Autodesk Fusion 360 part; units mm, degrees
(part 3 of 4)
  line L1469 (33.9941, -8.3096) -> (33.7624, -8.35)
  line L1470 (33.7624, -8.35) -> (33.6779, -8.255)
  line L1471 (33.6779, -8.255) -> (33.6779, -6.1823)
  line L1472 (5.5809, 13.4818) -> (5.5809, 13.4818)
  line L1473 (35.5029, -8.255) -> (35.5248, -6.0186)
  line L1474 (35.5248, -6.0186) -> (35.7566, -5.9782)
  line L1475 (35.7566, -5.9782) -> (35.8411, -6.0732)
  line L1476 (35.8411, -6.0732) -> (35.8411, -7.055)
  line L1477 (35.8411, -7.055) -> (36.8528, -7.055)
  line L1478 (36.8528, -7.055) -> (36.8747, -6.0186)
  line L1479 (36.8747, -6.0186) -> (37.1065, -5.9782)
  line L1480 (37.1065, -5.9782) -> (37.191, -6.0732)
  line L1481 (37.191, -6.0732) -> (37.1691, -8.3096)
  line L1482 (37.1691, -8.3096) -> (36.9374, -8.35)
  line L1483 (36.9374, -8.35) -> (36.8528, -8.255)
  line L1484 (36.8528, -8.255) -> (36.8528, -7.2732)
  line L1485 (36.8528, -7.2732) -> (35.8411, -7.2732)
  line L1486 (35.8411, -7.2732) -> (35.8192, -8.3096)
  line L1487 (35.8192, -8.3096) -> (35.5875, -8.35)
  line L1488 (35.5875, -8.35) -> (35.5029, -8.255)
  line L1489 (7.406, 11.4091) -> (7.406, 11.4091)
  line L1490 (38.9963, -7.375) -> (39.1977, -7.2732)
  line L1491 (39.1977, -7.2732) -> (39.2415, -7.1641)
  line L1492 (39.2415, -7.1641) -> (39.2304, -6.3429)
  line L1493 (39.2304, -6.3429) -> (39.1071, -6.2265)
  line L1494 (39.1071, -6.2265) -> (38.9033, -6.1823)
  line L1495 (38.9033, -6.1823) -> (38.3397, -6.1823)
  line L1496 (38.3397, -6.1823) -> (38.3178, -8.3096)
  line L1497 (38.3178, -8.3096) -> (38.0861, -8.35)
  line L1498 (38.0861, -8.35) -> (38.0015, -8.255)
  line L1499 (38.0015, -8.255) -> (38.0234, -6.0186)
  line L1500 (38.0234, -6.0186) -> (38.1706, -5.9641)
  line L1501 (38.1706, -5.9641) -> (39.0804, -5.9783)
  line L1502 (39.0804, -5.9783) -> (39.3126, -6.0531)
  line L1503 (39.3126, -6.0531) -> (39.4914, -6.1835)
  line L1504 (39.4914, -6.1835) -> (39.5576, -6.2862)
  line L1505 (39.5576, -6.2862) -> (39.5797, -6.4005)
  line L1506 (39.5797, -6.4005) -> (39.5742, -7.2226)
  line L1507 (39.5742, -7.2226) -> (39.5304, -7.3309)
  line L1508 (39.5304, -7.3309) -> (39.2528, -7.5386)
  line L1509 (39.2528, -7.5386) -> (39.684, -8.2877)
  line L1510 (39.684, -8.2877) -> (39.4726, -8.3605)
  line L1511 (39.4726, -8.3605) -> (39.3711, -8.3041)
  line L1512 (39.3711, -8.3041) -> (38.8709, -7.4657)
  line L1513 (38.8709, -7.4657) -> (38.9963, -7.375)
  line L1514 (10.8994, 12.2891) -> (10.8994, 12.2891)
  line L1515 (40.641, -8.255) -> (40.6629, -6.0186)
  line L1516 (40.6629, -6.0186) -> (40.8101, -5.9641)
  line L1517 (40.8101, -5.9641) -> (42.0036, -5.9959)
  line L1518 (42.0036, -5.9959) -> (42.0474, -6.1011)
  line L1519 (42.0474, -6.1011) -> (41.8838, -6.1823)
  line L1520 (41.8838, -6.1823) -> (40.9792, -6.1823)
  line L1521 (40.9792, -6.1823) -> (40.9792, -7.055)
  line L1522 (40.9792, -7.055) -> (41.8317, -7.0868)
  line L1523 (41.8317, -7.0868) -> (41.8755, -7.1929)
  line L1524 (41.8755, -7.1929) -> (41.7119, -7.2732)
  line L1525 (41.7119, -7.2732) -> (40.9792, -7.2732)
  line L1526 (40.9792, -7.2732) -> (40.9792, -8.1459)
  line L1527 (40.9792, -8.1459) -> (42.0036, -8.1777)
  line L1528 (42.0036, -8.1777) -> (42.0474, -8.2829)
  line L1529 (42.0474, -8.2829) -> (41.8838, -8.3641)
  line L1530 (41.8838, -8.3641) -> (40.6903, -8.3323)
  line L1531 (40.6903, -8.3323) -> (40.641, -8.255)
  line L1532 (12.544, 11.4091) -> (12.544, 11.4091)
  line L1533 (43.141, -8.255) -> (43.1629, -6.0186)
  line L1534 (43.1629, -6.0186) -> (43.3101, -5.9641)
  line L1535 (43.3101, -5.9641) -> (44.5036, -5.9959)
  line L1536 (44.5036, -5.9959) -> (44.5474, -6.1011)
  line L1537 (44.5474, -6.1011) -> (44.3838, -6.1823)
  line L1538 (44.3838, -6.1823) -> (43.4792, -6.1823)
  line L1539 (43.4792, -6.1823) -> (43.4792, -7.055)
  line L1540 (43.4792, -7.055) -> (44.3317, -7.0868)
  line L1541 (44.3317, -7.0868) -> (44.3755, -7.1929)
  line L1542 (44.3755, -7.1929) -> (44.2119, -7.2732)
  line L1543 (44.2119, -7.2732) -> (43.4792, -7.2732)
  line L1544 (43.4792, -7.2732) -> (43.4792, -8.1459)
  line L1545 (43.4792, -8.1459) -> (44.5036, -8.1777)
  line L1546 (44.5036, -8.1777) -> (44.5474, -8.2829)
  line L1547 (44.5474, -8.2829) -> (44.3838, -8.3641)
  line L1548 (44.3838, -8.3641) -> (43.1903, -8.3323)
  line L1549 (43.1903, -8.3323) -> (43.141, -8.255)
  line L1550 (15.044, 11.4091) -> (15.044, 11.4091)
  line L1551 (46.1751, -7.6132) -> (45.5068, -6.0444)
  line L1552 (45.5068, -6.0444) -> (45.6907, -5.965)
  line L1553 (45.6907, -5.965) -> (45.8284, -6.0368)
  line L1554 (45.8284, -6.0368) -> (46.347, -7.215)
  line L1555 (46.347, -7.215) -> (46.9106, -5.995)
  line L1556 (46.9106, -5.995) -> (47.1459, -5.9959)
  line L1557 (47.1459, -5.9959) -> (47.184, -6.1168)
  line L1558 (47.184, -6.1168) -> (46.5132, -7.615)
  line L1559 (46.5132, -7.615) -> (46.4913, -8.3096)
  line L1560 (46.4913, -8.3096) -> (46.2615, -8.35)
  line L1561 (46.2615, -8.35) -> (46.1751, -8.255)
  line L1562 (46.1751, -8.255) -> (46.1751, -7.6132)
  line L1563 (18.0781, 12.0509) -> (18.0781, 12.0509)
  line L1564 (48.4792, -7.055) -> (49.3317, -7.0868)
  line L1565 (49.3317, -7.0868) -> (49.3755, -7.1929)
  line L1566 (49.3755, -7.1929) -> (49.2119, -7.2732)
  line L1567 (49.2119, -7.2732) -> (48.4792, -7.2732)
  line L1568 (48.4792, -7.2732) -> (48.4573, -8.3096)
  line L1569 (48.4573, -8.3096) -> (48.2256, -8.35)
  line L1570 (48.2256, -8.35) -> (48.141, -8.255)
  line L1571 (48.141, -8.255) -> (48.1629, -6.0186)
  line L1572 (48.1629, -6.0186) -> (48.3101, -5.9641)
  line L1573 (48.3101, -5.9641) -> (49.5036, -5.9959)
  line L1574 (49.5036, -5.9959) -> (49.5474, -6.1011)
  line L1575 (49.5474, -6.1011) -> (49.3838, -6.1823)
  line L1576 (49.3838, -6.1823) -> (48.4792, -6.1823)
  line L1577 (48.4792, -6.1823) -> (48.4792, -7.055)
  line L1578 (20.3822, 12.6091) -> (20.3822, 12.6091)
  line L1579 (51.1779, -8.255) -> (51.1998, -6.0186)
  line L1580 (51.1998, -6.0186) -> (51.4315, -5.9782)
  line L1581 (51.4315, -5.9782) -> (51.5161, -6.0732)
  line L1582 (51.5161, -6.0732) -> (51.4941, -8.3096)
  line L1583 (51.4941, -8.3096) -> (51.2624, -8.35)
  line L1584 (51.2624, -8.35) -> (51.1779, -8.255)
  line L1585 (23.0809, 11.4091) -> (23.0809, 11.4091)
  line L1586 (53.4792, -7.055) -> (54.3317, -7.0868)
  line L1587 (54.3317, -7.0868) -> (54.3755, -7.1929)
  line L1588 (54.3755, -7.1929) -> (54.2119, -7.2732)
  line L1589 (54.2119, -7.2732) -> (53.4792, -7.2732)
  line L1590 (53.4792, -7.2732) -> (53.4573, -8.3096)
  line L1591 (53.4573, -8.3096) -> (53.2256, -8.35)
  line L1592 (53.2256, -8.35) -> (53.141, -8.255)
  line L1593 (53.141, -8.255) -> (53.1629, -6.0186)
  line L1594 (53.1629, -6.0186) -> (53.3101, -5.9641)
  line L1595 (53.3101, -5.9641) -> (54.5036, -5.9959)
  line L1596 (54.5036, -5.9959) -> (54.5474, -6.1011)
  line L1597 (54.5474, -6.1011) -> (54.3838, -6.1823)
  line L1598 (54.3838, -6.1823) -> (53.4792, -6.1823)
  line L1599 (53.4792, -6.1823) -> (53.4792, -7.055)
  line L1600 (25.3822, 12.6091) -> (25.3822, 12.6091)
  line L1601 (55.2789, -6.0968) -> (55.3424, -5.9862)
  line L1602 (55.3424, -5.9862) -> (55.6142, -6.055)
  line L1603 (55.6142, -6.055) -> (56.347, -7.8277)
  line L1604 (56.347, -7.8277) -> (57.1304, -5.995)
  line L1605 (57.1304, -5.995) -> (57.3686, -5.9959)
  line L1606 (57.3686, -5.9959) -> (57.4151, -6.0968)
  line L1607 (57.4151, -6.0968) -> (56.4681, -8.3314)
  line L1608 (56.4681, -8.3314) -> (56.1852, -8.2809)
  line L1609 (56.1852, -8.2809) -> (55.2789, -6.0968)
  line L1610 (27.1819, 13.5673) -> (27.1819, 13.5673)
  line L1611 (58.8892, -8.1459) -> (59.1257, -8.0853)
  line L1612 (59.1257, -8.0853) -> (59.2648, -7.9696)
  line L1613 (59.2648, -7.9696) -> (59.2979, -7.8586)
  line L1614 (59.2979, -7.8586) -> (59.2942, -6.4341)
  line L1615 (59.2942, -6.4341) -> (59.239, -6.3285)
  line L1616 (59.239, -6.3285) -> (59.0712, -6.2203)
  line L1617 (59.0712, -6.2203) -> (58.847, -6.1823)
  line L1618 (58.847, -6.1823) -> (58.3961, -6.1823)
  line L1619 (58.3961, -6.1823) -> (58.3741, -8.3096)
  line L1620 (58.3741, -8.3096) -> (58.1424, -8.35)
  line L1621 (58.1424, -8.35) -> (58.0579, -8.255)
  line L1622 (58.0579, -8.255) -> (58.0798, -6.0186)
  line L1623 (58.0798, -6.0186) -> (58.227, -5.9641)
  line L1624 (58.227, -5.9641) -> (58.9533, -5.9682)
  line L1625 (58.9533, -5.9682) -> (59.2403, -6.0304)
  line L1626 (59.2403, -6.0304) -> (59.4756, -6.1646)
  line L1627 (59.4756, -6.1646) -> (59.5783, -6.2777)
  line L1628 (59.5783, -6.2777) -> (59.6296, -6.4046)
  line L1629 (59.6296, -6.4046) -> (59.6296, -7.9272)
  line L1630 (59.6296, -7.9272) -> (59.5783, -8.0536)
  line L1631 (59.5783, -8.0536) -> (59.4756, -8.166)
  line L1632 (59.4756, -8.166) -> (59.259, -8.293)
  line L1633 (59.259, -8.293) -> (59.0073, -8.3565)
  line L1634 (59.0073, -8.3565) -> (58.7562, -8.3096)
  line L1635 (58.7562, -8.3096) -> (58.7568, -8.2009)
  line L1636 (58.7568, -8.2009) -> (58.8892, -8.1459)
  line L1637 (30.7923, 11.5182) -> (30.7923, 11.5182)
  line L1638 (30.641, -11.255) -> (30.6629, -9.0186)
  line L1639 (30.6629, -9.0186) -> (30.8101, -8.9641)
  line L1640 (30.8101, -8.9641) -> (32.0036, -8.9959)
  line L1641 (32.0036, -8.9959) -> (32.0474, -9.1011)
  line L1642 (32.0474, -9.1011) -> (31.8838, -9.1823)
  line L1643 (31.8838, -9.1823) -> (30.9792, -9.1823)
  line L1644 (30.9792, -9.1823) -> (30.9792, -10.055)
  line L1645 (30.9792, -10.055) -> (31.8317, -10.0868)
  line L1646 (31.8317, -10.0868) -> (31.8755, -10.1929)
  line L1647 (31.8755, -10.1929) -> (31.7119, -10.2732)
  line L1648 (31.7119, -10.2732) -> (30.9792, -10.2732)
  line L1649 (30.9792, -10.2732) -> (30.9792, -11.1459)
  line L1650 (30.9792, -11.1459) -> (32.0036, -11.1777)
  line L1651 (32.0036, -11.1777) -> (32.0474, -11.2829)
  line L1652 (32.0474, -11.2829) -> (31.8838, -11.3641)
  line L1653 (31.8838, -11.3641) -> (30.6903, -11.3323)
  line L1654 (30.6903, -11.3323) -> (30.641, -11.255)
  line L1655 (2.544, 8.4091) -> (2.544, 8.4091)
  line L1656 (33.6779, -11.255) -> (33.6998, -9.0186)
  line L1657 (33.6998, -9.0186) -> (33.9315, -8.9782)
  line L1658 (33.9315, -8.9782) -> (34.0161, -9.0732)
  line L1659 (34.0161, -9.0732) -> (33.9941, -11.3096)
  line L1660 (33.9941, -11.3096) -> (33.7624, -11.35)
  line L1661 (33.7624, -11.35) -> (33.6779, -11.255)
  line L1662 (5.5809, 8.4091) -> (5.5809, 8.4091)
  line L1663 (36.9045, -9.118) -> (36.9463, -9.2215)
  line L1664 (36.9463, -9.2215) -> (36.7415, -9.297)
  line L1665 (36.7415, -9.297) -> (36.4641, -9.1904)
  line L1666 (36.4641, -9.1904) -> (36.1753, -9.2017)
  line L1667 (36.1753, -9.2017) -> (35.9927, -9.2938)
  line L1668 (35.9927, -9.2938) -> (35.9175, -9.392)
  line L1669 (35.9175, -9.392) -> (35.9067, -10.9014)
  line L1670 (35.9067, -10.9014) -> (35.9604, -11.0054)
  line L1671 (35.9604, -11.0054) -> (36.1244, -11.1119)
  line L1672 (36.1244, -11.1119) -> (36.347, -11.1493)
  line L1673 (36.347, -11.1493) -> (36.7908, -11.1493)
  line L1674 (36.7908, -11.1493) -> (36.7908, -10.3261)
  line L1675 (36.7908, -10.3261) -> (36.4795, -10.2712)
  line L1676 (36.4795, -10.2712) -> (36.4795, -10.165)
  line L1677 (36.4795, -10.165) -> (36.6244, -10.1113)
  line L1678 (36.6244, -10.1113) -> (37.091, -10.1534)
  line L1679 (37.091, -10.1534) -> (37.1237, -10.2187)
  line L1680 (37.1237, -10.2187) -> (37.1021, -11.3092)
  line L1681 (37.1021, -11.3092) -> (36.9573, -11.3641)
  line L1682 (36.9573, -11.3641) -> (36.2423, -11.36)
  line L1683 (36.2423, -11.36) -> (35.9598, -11.2993)
  line L1684 (35.9598, -11.2993) -> (35.7282, -11.1679)
  line L1685 (35.7282, -11.1679) -> (35.6271, -11.0569)
  line L1686 (35.6271, -11.0569) -> (35.5766, -10.9323)
  line L1687 (35.5766, -10.9323) -> (35.5766, -9.3977)
  line L1688 (35.5766, -9.3977) -> (35.6271, -9.2728)
  line L1689 (35.6271, -9.2728) -> (35.7282, -9.1615)
  line L1690 (35.7282, -9.1615) -> (35.9598, -9.0293)
  line L1691 (35.9598, -9.0293) -> (36.2423, -8.9682)
  line L1692 (36.2423, -8.9682) -> (36.5519, -8.9812)
  line L1693 (36.5519, -8.9812) -> (36.9045, -9.118)
  line L1694 (8.8076, 10.5461) -> (8.8076, 10.5461)
  line L1695 (38.0029, -11.255) -> (38.0248, -9.0186)
  line L1696 (38.0248, -9.0186) -> (38.2566, -8.9782)
  line L1697 (38.2566, -8.9782) -> (38.3411, -9.0732)
  line L1698 (38.3411, -9.0732) -> (38.3411, -10.055)
  line L1699 (38.3411, -10.055) -> (39.3528, -10.055)
  line L1700 (39.3528, -10.055) -> (39.3747, -9.0186)
  line L1701 (39.3747, -9.0186) -> (39.6065, -8.9782)
  line L1702 (39.6065, -8.9782) -> (39.691, -9.0732)
  line L1703 (39.691, -9.0732) -> (39.6691, -11.3096)
  line L1704 (39.6691, -11.3096) -> (39.4374, -11.35)
  line L1705 (39.4374, -11.35) -> (39.3528, -11.255)
  line L1706 (39.3528, -11.255) -> (39.3528, -10.2732)
  line L1707 (39.3528, -10.2732) -> (38.3411, -10.2732)
  line L1708 (38.3411, -10.2732) -> (38.3192, -11.3096)
  line L1709 (38.3192, -11.3096) -> (38.0875, -11.35)
  line L1710 (38.0875, -11.35) -> (38.0029, -11.255)
  line L1711 (9.906, 8.4091) -> (9.906, 8.4091)
  line L1712 (41.1779, -9.1823) -> (40.5921, -9.1395)
  line L1713 (40.5921, -9.1395) -> (40.5702, -9.0311)
  line L1714 (40.5702, -9.0311) -> (40.727, -8.9641)
  line L1715 (40.727, -8.9641) -> (42.0867, -8.9959)
  line L1716 (42.0867, -8.9959) -> (42.1306, -9.102)
  line L1717 (42.1306, -9.102) -> (41.967, -9.1823)
  line L1718 (41.967, -9.1823) -> (41.5161, -9.1823)
  line L1719 (41.5161, -9.1823) -> (41.4941, -11.3096)
  line L1720 (41.4941, -11.3096) -> (41.2624, -11.35)
  line L1721 (41.2624, -11.35) -> (41.1779, -11.255)
  line L1722 (41.1779, -11.255) -> (41.1779, -9.1823)
  line L1723 (13.0809, 10.4818) -> (13.0809, 10.4818)
  line L1724 (45.3536, -9.0968) -> (44.5749, -11.3314)
  line L1725 (44.5749, -11.3314) -> (44.3768, -11.3414)
  line L1726 (44.3768, -11.3414) -> (44.3187, -11.2696)
  line L1727 (44.3187, -11.2696) -> (43.847, -9.895)
  line L1728 (43.847, -9.895) -> (43.3321, -11.3314)
  line L1729 (43.3321, -11.3314) -> (43.134, -11.3414)
  line L1730 (43.134, -11.3414) -> (43.0734, -11.2696)
  line L1731 (43.0734, -11.2696) -> (42.3489, -9.0311)
  line L1732 (42.3489, -9.0311) -> (42.549, -8.9718)
  line L1733 (42.549, -8.9718) -> (42.6422, -9.055)
  line L1734 (42.6422, -9.055) -> (43.2256, -10.7877)
  line L1735 (43.2256, -10.7877) -> (43.7442, -9.3568)
  line L1736 (43.7442, -9.3568) -> (43.9535, -9.3586)
  line L1737 (43.9535, -9.3586) -> (44.0093, -9.4368)
  line L1738 (44.0093, -9.4368) -> (44.4684, -10.7877)
  line L1739 (44.4684, -10.7877) -> (45.0974, -8.995)
  line L1740 (45.0974, -8.995) -> (45.3117, -8.9959)
  line L1741 (45.3117, -8.9959) -> (45.3536, -9.0968)
  line L1742 (17.2566, 10.5673) -> (17.2566, 10.5673)
  line L1743 (46.6117, -9.173) -> (46.5159, -9.0749)
  line L1744 (46.5159, -9.0749) -> (46.6403, -8.9694)
  line L1745 (46.6403, -8.9694) -> (46.9045, -9.0495)
  line L1746 (46.9045, -9.0495) -> (47.0328, -9.1557)
  line L1747 (47.0328, -9.1557) -> (47.1098, -9.2756)
  line L1748 (47.1098, -9.2756) -> (47.1355, -9.4092)
  line L1749 (47.1355, -9.4092) -> (47.129, -10.9875)
  line L1750 (47.129, -10.9875) -> (47.0777, -11.1143)
  line L1751 (47.0777, -11.1143) -> (46.9751, -11.2273)
  line L1752 (46.9751, -11.2273) -> (46.662, -11.3632)
  line L1753 (46.662, -11.3632) -> (46.5173, -11.2693)
  line L1754 (46.5173, -11.2693) -> (46.7644, -11.0303)
  line L1755 (46.7644, -11.0303) -> (46.7975, -10.919)
  line L1756 (46.7975, -10.919) -> (46.7939, -9.3702)
  line L1757 (46.7939, -9.3702) -> (46.7387, -9.2647)
  line L1758 (46.7387, -9.2647) -> (46.6117, -9.173)
  line L1759 (18.5147, 10.4911) -> (18.5147, 10.4911)
  line L1760 (45.9105, -8.9841) -> (46.1561, -9.0198)
  line L1761 (46.1561, -9.0198) -> (46.1567, -9.1272)
  line L1762 (46.1567, -9.1272) -> (45.9552, -9.2647)
  line L1763 (45.9552, -9.2647) -> (45.9001, -9.3702)
  line L1764 (45.9001, -9.3702) -> (45.9001, -10.958)
  line L1765 (45.9001, -10.958) -> (45.9552, -11.0635)
  line L1766 (45.9552, -11.0635) -> (46.1766, -11.2385)
  line L1767 (46.1766, -11.2385) -> (46.0916, -11.3482)
  line L1768 (46.0916, -11.3482) -> (45.7894, -11.2787)
  line L1769 (45.7894, -11.2787) -> (45.6611, -11.1725)
  line L1770 (45.6611, -11.1725) -> (45.5841, -11.0526)
  line L1771 (45.5841, -11.0526) -> (45.5585, -10.919)
  line L1772 (45.5585, -10.919) -> (45.5649, -9.3407)
  line L1773 (45.5649, -9.3407) -> (45.6162, -9.2139)
  line L1774 (45.6162, -9.2139) -> (45.7188, -9.1009)
  line L1775 (45.7188, -9.1009) -> (45.9105, -8.9841)
  line L1776 (17.8135, 10.68) -> (17.8135, 10.68)
  line L1777 (48.2238, -11.2001) -> (48.1749, -11.1029)
  line L1778 (48.1749, -11.1029) -> (48.344, -11.0167)
  line L1779 (48.344, -11.0167) -> (48.7119, -11.1462)
  line L1780 (48.7119, -11.1462) -> (48.9964, -11.1178)
  line L1781 (48.9964, -11.1178) -> (49.1604, -11.0206)
  line L1782 (49.1604, -11.0206) -> (49.2296, -10.8598)
  line L1783 (49.2296, -10.8598) -> (49.2144, -10.76)
  line L1784 (49.2144, -10.76) -> (49.0923, -10.5437)
  line L1785 (49.0923, -10.5437) -> (48.8481, -10.305)
  line L1786 (48.8481, -10.305) -> (48.5132, -10.0492)
  line L1787 (48.5132, -10.0492) -> (48.2702, -9.8035)
  line L1788 (48.2702, -9.8035) -> (48.1488, -9.5719)
  line L1789 (48.1488, -9.5719) -> (48.1336, -9.4332)
  line L1790 (48.1336, -9.4332) -> (48.1703, -9.3033)
  line L1791 (48.1703, -9.3033) -> (48.2551, -9.1886)
  line L1792 (48.2551, -9.1886) -> (48.4626, -9.051)
  line L1793 (48.4626, -9.051) -> (48.7097, -8.978)
  line L1794 (48.7097, -8.978) -> (49.0426, -8.9715)
  line L1795 (49.0426, -8.9715) -> (49.3153, -9.0409)
  line L1796 (49.3153, -9.0409) -> (49.5179, -9.1947)
  line L1797 (49.5179, -9.1947) -> (49.3954, -9.3066)
  line L1798 (49.3954, -9.3066) -> (49.035, -9.19)
  line L1799 (49.035, -9.19) -> (48.739, -9.1951)
  line L1800 (48.739, -9.1951) -> (48.5652, -9.2755)
  line L1801 (48.5652, -9.2755) -> (48.4825, -9.3703)
  line L1802 (48.4825, -9.3703) -> (48.4616, -9.4596)
  line L1803 (48.4616, -9.4596) -> (48.5232, -9.6395)
  line L1804 (48.5232, -9.6395) -> (48.7082, -9.8523)
  line L1805 (48.7082, -9.8523) -> (49.1826, -10.2267)
  line L1806 (49.1826, -10.2267) -> (49.4244, -10.4811)
  line L1807 (49.4244, -10.4811) -> (49.5452, -10.7311)
  line L1808 (49.5452, -10.7311) -> (49.5576, -10.8933)
  line L1809 (49.5576, -10.8933) -> (49.5209, -11.0232)
  line L1810 (49.5209, -11.0232) -> (49.4361, -11.1378)
  line L1811 (49.4361, -11.1378) -> (49.2286, -11.2759)
  line L1812 (49.2286, -11.2759) -> (48.9803, -11.35)
  line L1813 (48.9803, -11.35) -> (48.6486, -11.3561)
  line L1814 (48.6486, -11.3561) -> (48.3759, -11.2857)
  line L1815 (48.3759, -11.2857) -> (48.2238, -11.2001)
  line L1816 (20.1268, 8.464) -> (20.1268, 8.464)
  line L1817 (51.1779, -11.255) -> (51.1998, -9.0186)
  line L1818 (51.1998, -9.0186) -> (51.4315, -8.9782)
  line L1819 (51.4315, -8.9782) -> (51.5161, -9.0732)
  line L1820 (51.5161, -9.0732) -> (51.4941, -11.3096)
  line L1821 (51.4941, -11.3096) -> (51.2624, -11.35)
  line L1822 (51.2624, -11.35) -> (51.1779, -11.255)
  line L1823 (23.0809, 8.4091) -> (23.0809, 8.4091)
  line L1824 (53.2312, -9.0241) -> (53.8484, -9.8986)
  line L1825 (53.8484, -9.8986) -> (54.5229, -8.9821)
  line L1826 (54.5229, -8.9821) -> (54.7561, -9.0132)
  line L1827 (54.7561, -9.0132) -> (54.7643, -9.1223)
  line L1828 (54.7643, -9.1223) -> (54.0316, -10.1641)
  line L1829 (54.0316, -10.1641) -> (54.7756, -11.2877)
  line L1830 (54.7756, -11.2877) -> (54.5642, -11.3586)
  line L1831 (54.5642, -11.3586) -> (54.4627, -11.3041)
  line L1832 (54.4627, -11.3041) -> (53.8484, -10.4296)
  line L1833 (53.8484, -10.4296) -> (53.1736, -11.3461)
  line L1834 (53.1736, -11.3461) -> (52.9406, -11.3142)
  line L1835 (52.9406, -11.3142) -> (52.9296, -11.2059)
  line L1836 (52.9296, -11.2059) -> (53.6624, -10.1641)
  line L1837 (53.6624, -10.1641) -> (52.9184, -9.0386)
  line L1838 (52.9184, -9.0386) -> (53.1297, -8.9696)
  line L1839 (53.1297, -8.9696) -> (53.2312, -9.0241)
  line L1840 (25.1342, 10.64) -> (25.1342, 10.64)
  line L1841 (55.641, -11.255) -> (55.6629, -9.0186)
  line L1842 (55.6629, -9.0186) -> (55.8101, -8.9641)
  line L1843 (55.8101, -8.9641) -> (57.0036, -8.9959)
  line L1844 (57.0036, -8.9959) -> (57.0474, -9.1011)
  line L1845 (57.0474, -9.1011) -> (56.8838, -9.1823)
  line L1846 (56.8838, -9.1823) -> (55.9792, -9.1823)
  line L1847 (55.9792, -9.1823) -> (55.9792, -10.055)
  line L1848 (55.9792, -10.055) -> (56.8317, -10.0868)
  line L1849 (56.8317, -10.0868) -> (56.8755, -10.1929)
  line L1850 (56.8755, -10.1929) -> (56.7119, -10.2732)
  line L1851 (56.7119, -10.2732) -> (55.9792, -10.2732)
  line L1852 (55.9792, -10.2732) -> (55.9792, -11.1459)
  line L1853 (55.9792, -11.1459) -> (57.0036, -11.1777)
  line L1854 (57.0036, -11.1777) -> (57.0474, -11.2829)
  line L1855 (57.0474, -11.2829) -> (56.8838, -11.3641)
  line L1856 (56.8838, -11.3641) -> (55.6903, -11.3323)
  line L1857 (55.6903, -11.3323) -> (55.641, -11.255)
  line L1858 (27.544, 8.4091) -> (27.544, 8.4091)
  line L1859 (58.9963, -10.375) -> (59.1977, -10.2732)
  line L1860 (59.1977, -10.2732) -> (59.2415, -10.1641)
  line L1861 (59.2415, -10.1641) -> (59.2304, -9.3429)
  line L1862 (59.2304, -9.3429) -> (59.1071, -9.2265)
  line L1863 (59.1071, -9.2265) -> (58.9033, -9.1823)
  line L1864 (58.9033, -9.1823) -> (58.3397, -9.1823)
  line L1865 (58.3397, -9.1823) -> (58.3178, -11.3096)
  line L1866 (58.3178, -11.3096) -> (58.0861, -11.35)
  line L1867 (58.0861, -11.35) -> (58.0015, -11.255)
  line L1868 (58.0015, -11.255) -> (58.0234, -9.0186)
  line L1869 (58.0234, -9.0186) -> (58.1706, -8.9641)
  line L1870 (58.1706, -8.9641) -> (59.0804, -8.9783)
  line L1871 (59.0804, -8.9783) -> (59.3126, -9.0531)
  line L1872 (59.3126, -9.0531) -> (59.4914, -9.1835)
  line L1873 (59.4914, -9.1835) -> (59.5576, -9.2862)
  line L1874 (59.5576, -9.2862) -> (59.5797, -9.4005)
  line L1875 (59.5797, -9.4005) -> (59.5742, -10.2226)
  line L1876 (59.5742, -10.2226) -> (59.5304, -10.3309)
  line L1877 (59.5304, -10.3309) -> (59.2528, -10.5386)
  line L1878 (59.2528, -10.5386) -> (59.684, -11.2877)
  line L1879 (59.684, -11.2877) -> (59.4726, -11.3605)
  line L1880 (59.4726, -11.3605) -> (59.3711, -11.3041)
  line L1881 (59.3711, -11.3041) -> (58.8709, -10.4657)
  line L1882 (58.8709, -10.4657) -> (58.9963, -10.375)
  line L1883 (30.8994, 9.2891) -> (30.8994, 9.2891)
  line L1884 (31.6117, -12.173) -> (31.5159, -12.0749)
  line L1885 (31.5159, -12.0749) -> (31.6403, -11.9694)
  line L1886 (31.6403, -11.9694) -> (31.9045, -12.0495)
  line L1887 (31.9045, -12.0495) -> (32.0328, -12.1557)
  line L1888 (32.0328, -12.1557) -> (32.1098, -12.2756)
  line L1889 (32.1098, -12.2756) -> (32.1355, -12.4092)
  line L1890 (32.1355, -12.4092) -> (32.129, -13.9875)
  line L1891 (32.129, -13.9875) -> (32.0777, -14.1143)
  line L1892 (32.0777, -14.1143) -> (31.9751, -14.2273)
  line L1893 (31.9751, -14.2273) -> (31.662, -14.3632)
  line L1894 (31.662, -14.3632) -> (31.5173, -14.2693)
  line L1895 (31.5173, -14.2693) -> (31.7644, -14.0303)
  line L1896 (31.7644, -14.0303) -> (31.7975, -13.919)
  line L1897 (31.7975, -13.919) -> (31.7939, -12.3702)
  line L1898 (31.7939, -12.3702) -> (31.7387, -12.2647)
  line L1899 (31.7387, -12.2647) -> (31.6117, -12.173)
  line L1900 (3.5147, 7.4911) -> (3.5147, 7.4911)
  line L1901 (30.9105, -11.9841) -> (31.1561, -12.0198)
  line L1902 (31.1561, -12.0198) -> (31.1567, -12.1272)
  line L1903 (31.1567, -12.1272) -> (30.9552, -12.2647)
  line L1904 (30.9552, -12.2647) -> (30.9001, -12.3702)
  line L1905 (30.9001, -12.3702) -> (30.9001, -13.958)
  line L1906 (30.9001, -13.958) -> (30.9552, -14.0635)
  line L1907 (30.9552, -14.0635) -> (31.1766, -14.2385)
  line L1908 (31.1766, -14.2385) -> (31.0916, -14.3482)
  line L1909 (31.0916, -14.3482) -> (30.7894, -14.2787)
  line L1910 (30.7894, -14.2787) -> (30.6611, -14.1725)
  line L1911 (30.6611, -14.1725) -> (30.5841, -14.0526)
  line L1912 (30.5841, -14.0526) -> (30.5585, -13.919)
  line L1913 (30.5585, -13.919) -> (30.5649, -12.3407)
  line L1914 (30.5649, -12.3407) -> (30.6162, -12.2139)
  line L1915 (30.6162, -12.2139) -> (30.7188, -12.1009)
  line L1916 (30.7188, -12.1009) -> (30.9105, -11.9841)
  line L1917 (2.8135, 7.68) -> (2.8135, 7.68)
  line L1918 (33.2274, -12.5527) -> (33.2055, -14.3096)
  line L1919 (33.2055, -14.3096) -> (32.974, -14.35)
  line L1920 (32.974, -14.35) -> (32.8895, -14.2551)
  line L1921 (32.8895, -14.2551) -> (32.9114, -12.0186)
  line L1922 (32.9114, -12.0186) -> (33.1436, -11.9778)
  line L1923 (33.1436, -11.9778) -> (33.2077, -12.0204)
  line L1924 (33.2077, -12.0204) -> (34.4665, -13.7664)
  line L1925 (34.4665, -13.7664) -> (34.4884, -12.0186)
  line L1926 (34.4884, -12.0186) -> (34.7199, -11.9782)
  line L1927 (34.7199, -11.9782) -> (34.8044, -12.0731)
  line L1928 (34.8044, -12.0731) -> (34.7831, -14.3094)
  line L1929 (34.7831, -14.3094) -> (34.5516, -14.3496)
  line L1930 (34.5516, -14.3496) -> (34.4749, -14.2914)
  line L1931 (34.4749, -14.2914) -> (33.2274, -12.5527)
  line L1932 (5.1305, 7.1114) -> (5.1305, 7.1114)
  line L1933 (35.641, -14.255) -> (35.6629, -12.0186)
  line L1934 (35.6629, -12.0186) -> (35.8101, -11.9641)
  line L1935 (35.8101, -11.9641) -> (37.0036, -11.9959)
  line L1936 (37.0036, -11.9959) -> (37.0474, -12.1011)
  line L1937 (37.0474, -12.1011) -> (36.8838, -12.1823)
  line L1938 (36.8838, -12.1823) -> (35.9792, -12.1823)
  line L1939 (35.9792, -12.1823) -> (35.9792, -13.055)
  line L1940 (35.9792, -13.055) -> (36.8317, -13.0868)
  line L1941 (36.8317, -13.0868) -> (36.8755, -13.1929)
  line L1942 (36.8755, -13.1929) -> (36.7119, -13.2732)
  line L1943 (36.7119, -13.2732) -> (35.9792, -13.2732)
  line L1944 (35.9792, -13.2732) -> (35.9792, -14.1459)
  line L1945 (35.9792, -14.1459) -> (37.0036, -14.1777)
  line L1946 (37.0036, -14.1777) -> (37.0474, -14.2829)
  line L1947 (37.0474, -14.2829) -> (36.8838, -14.3641)
  line L1948 (36.8838, -14.3641) -> (35.6903, -14.3323)
  line L1949 (35.6903, -14.3323) -> (35.641, -14.255)
  line L1950 (7.544, 5.4091) -> (7.544, 5.4091)
  line L1951 (38.6779, -12.1823) -> (38.0921, -12.1395)
  line L1952 (38.0921, -12.1395) -> (38.0702, -12.0311)
  line L1953 (38.0702, -12.0311) -> (38.227, -11.9641)
  line L1954 (38.227, -11.9641) -> (39.5867, -11.9959)
  line L1955 (39.5867, -11.9959) -> (39.6306, -12.102)
  line L1956 (39.6306, -12.102) -> (39.467, -12.1823)
  line L1957 (39.467, -12.1823) -> (39.0161, -12.1823)
  line L1958 (39.0161, -12.1823) -> (38.9941, -14.3096)
  line L1959 (38.9941, -14.3096) -> (38.7624, -14.35)
  line L1960 (38.7624, -14.35) -> (38.6779, -14.255)
  line L1961 (38.6779, -14.255) -> (38.6779, -12.1823)
  line L1962 (10.5809, 7.4818) -> (10.5809, 7.4818)
  line L1963 (40.641, -14.255) -> (40.6629, -12.0186)
  line L1964 (40.6629, -12.0186) -> (40.8101, -11.9641)
  line L1965 (40.8101, -11.9641) -> (42.0036, -11.9959)
  line L1966 (42.0036, -11.9959) -> (42.0474, -12.1011)
  line L1967 (42.0474, -12.1011) -> (41.8838, -12.1823)
  line L1968 (41.8838, -12.1823) -> (40.9792, -12.1823)
  line L1969 (40.9792, -12.1823) -> (40.9792, -13.055)
  line L1970 (40.9792, -13.055) -> (41.8317, -13.0868)
  line L1971 (41.8317, -13.0868) -> (41.8755, -13.1929)
  line L1972 (41.8755, -13.1929) -> (41.7119, -13.2732)
  line L1973 (41.7119, -13.2732) -> (40.9792, -13.2732)
  line L1974 (40.9792, -13.2732) -> (40.9792, -14.1459)
  line L1975 (40.9792, -14.1459) -> (42.0036, -14.1777)
  line L1976 (42.0036, -14.1777) -> (42.0474, -14.2829)
  line L1977 (42.0474, -14.2829) -> (41.8838, -14.3641)
  line L1978 (41.8838, -14.3641) -> (40.6903, -14.3323)
  line L1979 (40.6903, -14.3323) -> (40.641, -14.255)
  line L1980 (12.544, 5.4091) -> (12.544, 5.4091)
  line L1981 (43.2274, -12.5527) -> (43.2055, -14.3096)
  line L1982 (43.2055, -14.3096) -> (42.974, -14.35)
  line L1983 (42.974, -14.35) -> (42.8895, -14.2551)
  line L1984 (42.8895, -14.2551) -> (42.9114, -12.0186)
  line L1985 (42.9114, -12.0186) -> (43.1436, -11.9778)
  line L1986 (43.1436, -11.9778) -> (43.2077, -12.0204)
  line L1987 (43.2077, -12.0204) -> (44.4665, -13.7664)
  line L1988 (44.4665, -13.7664) -> (44.4884, -12.0186)
  line L1989 (44.4884, -12.0186) -> (44.7199, -11.9782)
  line L1990 (44.7199, -11.9782) -> (44.8044, -12.0731)
  line L1991 (44.8044, -12.0731) -> (44.7831, -14.3094)
  line L1992 (44.7831, -14.3094) -> (44.5516, -14.3496)
  line L1993 (44.5516, -14.3496) -> (44.4749, -14.2914)
  line L1994 (44.4749, -14.2914) -> (43.2274, -12.5527)
  line L1995 (15.1305, 7.1114) -> (15.1305, 7.1114)
  line L1996 (45.9792, -13.055) -> (46.8317, -13.0868)
  line L1997 (46.8317, -13.0868) -> (46.8755, -13.1929)
  line L1998 (46.8755, -13.1929) -> (46.7119, -13.2732)
  line L1999 (46.7119, -13.2732) -> (45.9792, -13.2732)
  line L2000 (45.9792, -13.2732) -> (45.9573, -14.3096)
  line L2001 (45.9573, -14.3096) -> (45.7256, -14.35)
  line L2002 (45.7256, -14.35) -> (45.641, -14.255)
  line L2003 (45.641, -14.255) -> (45.6629, -12.0186)
  line L2004 (45.6629, -12.0186) -> (45.8101, -11.9641)
  line L2005 (45.8101, -11.9641) -> (47.0036, -11.9959)
  line L2006 (47.0036, -11.9959) -> (47.0474, -12.1011)
  line L2007 (47.0474, -12.1011) -> (46.8838, -12.1823)
  line L2008 (46.8838, -12.1823) -> (45.9792, -12.1823)
  line L2009 (45.9792, -12.1823) -> (45.9792, -13.055)
  line L2010 (17.8822, 6.6091) -> (17.8822, 6.6091)
  line L2011 (48.6779, -14.255) -> (48.6998, -12.0186)
  line L2012 (48.6998, -12.0186) -> (48.9315, -11.9782)
  line L2013 (48.9315, -11.9782) -> (49.0161, -12.0732)
  line L2014 (49.0161, -12.0732) -> (48.9941, -14.3096)
  line L2015 (48.9941, -14.3096) -> (48.7624, -14.35)
  line L2016 (48.7624, -14.35) -> (48.6779, -14.255)
  line L2017 (20.5809, 5.4091) -> (20.5809, 5.4091)
  line L2018 (50.2789, -12.0968) -> (50.3424, -11.9862)
  line L2019 (50.3424, -11.9862) -> (50.6142, -12.055)
  line L2020 (50.6142, -12.055) -> (51.347, -13.8277)
  line L2021 (51.347, -13.8277) -> (52.1304, -11.995)
  line L2022 (52.1304, -11.995) -> (52.3686, -11.9959)
  line L2023 (52.3686, -11.9959) -> (52.4151, -12.0968)
  line L2024 (52.4151, -12.0968) -> (51.4681, -14.3314)
  line L2025 (51.4681, -14.3314) -> (51.246, -14.3414)
  line L2026 (51.246, -14.3414) -> (51.1807, -14.2696)
  line L2027 (51.1807, -14.2696) -> (50.2789, -12.0968)
  line L2028 (22.1819, 7.5673) -> (22.1819, 7.5673)
  line L2029 (53.141, -14.255) -> (53.1629, -12.0186)
  line L2030 (53.1629, -12.0186) -> (53.3101, -11.9641)
  line L2031 (53.3101, -11.9641) -> (54.5036, -11.9959)
  line L2032 (54.5036, -11.9959) -> (54.5474, -12.1011)
  line L2033 (54.5474, -12.1011) -> (54.3838, -12.1823)
  line L2034 (54.3838, -12.1823) -> (53.4792, -12.1823)
  line L2035 (53.4792, -12.1823) -> (53.4792, -13.055)
  line L2036 (53.4792, -13.055) -> (54.3317, -13.0868)
  line L2037 (54.3317, -13.0868) -> (54.3755, -13.1929)
  line L2038 (54.3755, -13.1929) -> (54.2119, -13.2732)
  line L2039 (54.2119, -13.2732) -> (53.4792, -13.2732)
  line L2040 (53.4792, -13.2732) -> (53.4792, -14.1459)
  line L2041 (53.4792, -14.1459) -> (54.5036, -14.1777)
  line L2042 (54.5036, -14.1777) -> (54.5474, -14.2829)
  line L2043 (54.5474, -14.2829) -> (54.3838, -14.3641)
  line L2044 (54.3838, -14.3641) -> (53.1903, -14.3323)
  line L2045 (53.1903, -14.3323) -> (53.141, -14.255)
  line L2046 (25.044, 5.4091) -> (25.044, 5.4091)
  line L2047 (55.7238, -14.2001) -> (55.6749, -14.1029)
  line L2048 (55.6749, -14.1029) -> (55.844, -14.0167)
  line L2049 (55.844, -14.0167) -> (56.2119, -14.1462)
  line L2050 (56.2119, -14.1462) -> (56.4964, -14.1178)
  line L2051 (56.4964, -14.1178) -> (56.6604, -14.0206)
  line L2052 (56.6604, -14.0206) -> (56.7296, -13.8598)
  line L2053 (56.7296, -13.8598) -> (56.7144, -13.76)
  line L2054 (56.7144, -13.76) -> (56.5923, -13.5437)
  line L2055 (56.5923, -13.5437) -> (56.3481, -13.305)
  line L2056 (56.3481, -13.305) -> (56.0132, -13.0492)
  line L2057 (56.0132, -13.0492) -> (55.7702, -12.8035)
  line L2058 (55.7702, -12.8035) -> (55.6488, -12.5719)
  line L2059 (55.6488, -12.5719) -> (55.6336, -12.4332)
  line L2060 (55.6336, -12.4332) -> (55.6703, -12.3033)
  line L2061 (55.6703, -12.3033) -> (55.7551, -12.1886)
  line L2062 (55.7551, -12.1886) -> (55.9626, -12.051)
  line L2063 (55.9626, -12.051) -> (56.2097, -11.978)
  line L2064 (56.2097, -11.978) -> (56.5426, -11.9715)
  line L2065 (56.5426, -11.9715) -> (56.8153, -12.0409)
  line L2066 (56.8153, -12.0409) -> (57.0179, -12.1947)
  line L2067 (57.0179, -12.1947) -> (56.8954, -12.3066)
  line L2068 (56.8954, -12.3066) -> (56.535, -12.19)
  line L2069 (56.535, -12.19) -> (56.239, -12.1951)
  line L2070 (56.239, -12.1951) -> (56.0652, -12.2755)
  line L2071 (56.0652, -12.2755) -> (55.9825, -12.3703)
  line L2072 (55.9825, -12.3703) -> (55.9616, -12.4596)
  line L2073 (55.9616, -12.4596) -> (56.0232, -12.6395)
  line L2074 (56.0232, -12.6395) -> (56.2082, -12.8523)
  line L2075 (56.2082, -12.8523) -> (56.6826, -13.2267)
  line L2076 (56.6826, -13.2267) -> (56.9244, -13.4811)
  line L2077 (56.9244, -13.4811) -> (57.0452, -13.7311)
  line L2078 (57.0452, -13.7311) -> (57.0576, -13.8933)
  line L2079 (57.0576, -13.8933) -> (57.0209, -14.0232)
  line L2080 (57.0209, -14.0232) -> (56.9361, -14.1378)
  line L2081 (56.9361, -14.1378) -> (56.7286, -14.2759)
  line L2082 (56.7286, -14.2759) -> (56.4803, -14.35)
  line L2083 (56.4803, -14.35) -> (56.1486, -14.3561)
  line L2084 (56.1486, -14.3561) -> (55.8759, -14.2857)
  line L2085 (55.8759, -14.2857) -> (55.7238, -14.2001)
  line L2086 (27.6268, 5.464) -> (27.6268, 5.464)
  line L2087 (58.141, -14.255) -> (58.1629, -12.0186)
  line L2088 (58.1629, -12.0186) -> (58.3101, -11.9641)
  line L2089 (58.3101, -11.9641) -> (59.5036, -11.9959)
  line L2090 (59.5036, -11.9959) -> (59.5474, -12.1011)
  line L2091 (59.5474, -12.1011) -> (59.3838, -12.1823)
  line L2092 (59.3838, -12.1823) -> (58.4792, -12.1823)
  line L2093 (58.4792, -12.1823) -> (58.4792, -13.055)
  line L2094 (58.4792, -13.055) -> (59.3317, -13.0868)
  line L2095 (59.3317, -13.0868) -> (59.3755, -13.1929)
  line L2096 (59.3755, -13.1929) -> (59.2119, -13.2732)
  line L2097 (59.2119, -13.2732) -> (58.4792, -13.2732)
  line L2098 (58.4792, -13.2732) -> (58.4792, -14.1459)
  line L2099 (58.4792, -14.1459) -> (59.5036, -14.1777)
  line L2100 (59.5036, -14.1777) -> (59.5474, -14.2829)
  line L2101 (59.5474, -14.2829) -> (59.3838, -14.3641)
  line L2102 (59.3838, -14.3641) -> (58.1903, -14.3323)
  line L2103 (58.1903, -14.3323) -> (58.141, -14.255)
  line L2104 (30.044, 5.4091) -> (30.044, 5.4091)
  line L2105 (30.5029, -17.255) -> (30.5248, -15.0186)
  line L2106 (30.5248, -15.0186) -> (30.7566, -14.9782)
  line L2107 (30.7566, -14.9782) -> (30.8411, -15.0732)
  line L2108 (30.8411, -15.0732) -> (30.8411, -16.055)
  line L2109 (30.8411, -16.055) -> (31.8528, -16.055)
  line L2110 (31.8528, -16.055) -> (31.8747, -15.0186)
  line L2111 (31.8747, -15.0186) -> (32.1065, -14.9782)
  line L2112 (32.1065, -14.9782) -> (32.191, -15.0732)
  line L2113 (32.191, -15.0732) -> (32.1691, -17.3096)
  line L2114 (32.1691, -17.3096) -> (31.9374, -17.35)
  line L2115 (31.9374, -17.35) -> (31.8528, -17.255)
  line L2116 (31.8528, -17.255) -> (31.8528, -16.2732)
  line L2117 (31.8528, -16.2732) -> (30.8411, -16.2732)
  line L2118 (30.8411, -16.2732) -> (30.8192, -17.3096)
  line L2119 (30.8192, -17.3096) -> (30.5875, -17.35)
  line L2120 (30.5875, -17.35) -> (30.5029, -17.255)
  line L2121 (2.406, 2.4091) -> (2.406, 2.4091)
  line L2122 (33.2238, -17.2001) -> (33.1749, -17.1029)
  line L2123 (33.1749, -17.1029) -> (33.344, -17.0167)
  line L2124 (33.344, -17.0167) -> (33.7119, -17.1462)
  line L2125 (33.7119, -17.1462) -> (33.9964, -17.1178)
  line L2126 (33.9964, -17.1178) -> (34.1604, -17.0206)
  line L2127 (34.1604, -17.0206) -> (34.2296, -16.8598)
  line L2128 (34.2296, -16.8598) -> (34.2144, -16.76)
  line L2129 (34.2144, -16.76) -> (34.0923, -16.5437)
  line L2130 (34.0923, -16.5437) -> (33.8481, -16.305)
  line L2131 (33.8481, -16.305) -> (33.5132, -16.0492)
  line L2132 (33.5132, -16.0492) -> (33.2702, -15.8035)
  line L2133 (33.2702, -15.8035) -> (33.1488, -15.5719)
  line L2134 (33.1488, -15.5719) -> (33.1336, -15.4332)
  line L2135 (33.1336, -15.4332) -> (33.1703, -15.3033)
  line L2136 (33.1703, -15.3033) -> (33.2551, -15.1886)
  line L2137 (33.2551, -15.1886) -> (33.4626, -15.051)
  line L2138 (33.4626, -15.051) -> (33.7097, -14.978)
  line L2139 (33.7097, -14.978) -> (34.0426, -14.9715)
  line L2140 (34.0426, -14.9715) -> (34.3153, -15.0409)
  line L2141 (34.3153, -15.0409) -> (34.5179, -15.1947)
  line L2142 (34.5179, -15.1947) -> (34.3954, -15.3066)
  line L2143 (34.3954, -15.3066) -> (34.035, -15.19)
  line L2144 (34.035, -15.19) -> (33.739, -15.1951)
  line L2145 (33.739, -15.1951) -> (33.5652, -15.2755)
  line L2146 (33.5652, -15.2755) -> (33.4825, -15.3703)
  line L2147 (33.4825, -15.3703) -> (33.4616, -15.4596)
  line L2148 (33.4616, -15.4596) -> (33.5232, -15.6395)
  line L2149 (33.5232, -15.6395) -> (33.7082, -15.8523)
  line L2150 (33.7082, -15.8523) -> (34.1826, -16.2267)
  line L2151 (34.1826, -16.2267) -> (34.4244, -16.4811)
  line L2152 (34.4244, -16.4811) -> (34.5452, -16.7311)
  line L2153 (34.5452, -16.7311) -> (34.5576, -16.8933)
  line L2154 (34.5576, -16.8933) -> (34.5209, -17.0232)
  line L2155 (34.5209, -17.0232) -> (34.4361, -17.1378)
  line L2156 (34.4361, -17.1378) -> (34.2286, -17.2759)
  line L2157 (34.2286, -17.2759) -> (33.9803, -17.35)
  line L2158 (33.9803, -17.35) -> (33.6486, -17.3561)
  line L2159 (33.6486, -17.3561) -> (33.3759, -17.2857)
  line L2160 (33.3759, -17.2857) -> (33.2238, -17.2001)
  line L2161 (5.1268, 2.464) -> (5.1268, 2.464)
  line L2162 (35.641, -17.255) -> (35.6629, -15.0186)
  line L2163 (35.6629, -15.0186) -> (35.8101, -14.9641)
  line L2164 (35.8101, -14.9641) -> (37.0036, -14.9959)
  line L2165 (37.0036, -14.9959) -> (37.0474, -15.1011)
  line L2166 (37.0474, -15.1011) -> (36.8838, -15.1823)
  line L2167 (36.8838, -15.1823) -> (35.9792, -15.1823)
  line L2168 (35.9792, -15.1823) -> (35.9792, -16.055)
  line L2169 (35.9792, -16.055) -> (36.8317, -16.0868)
  line L2170 (36.8317, -16.0868) -> (36.8755, -16.1929)
  line L2171 (36.8755, -16.1929) -> (36.7119, -16.2732)
  line L2172 (36.7119, -16.2732) -> (35.9792, -16.2732)
  line L2173 (35.9792, -16.2732) -> (35.9792, -17.1459)
  line L2174 (35.9792, -17.1459) -> (37.0036, -17.1777)
  line L2175 (37.0036, -17.1777) -> (37.0474, -17.2829)
  line L2176 (37.0474, -17.2829) -> (36.8838, -17.3641)
  line L2177 (36.8838, -17.3641) -> (35.6903, -17.3323)
  line L2178 (35.6903, -17.3323) -> (35.641, -17.255)
  line L2179 (7.544, 2.4091) -> (7.544, 2.4091)
  line L2180 (37.7789, -15.0968) -> (37.8424, -14.9862)
  line L2181 (37.8424, -14.9862) -> (38.1142, -15.055)
  line L2182 (38.1142, -15.055) -> (38.847, -16.8277)
  line L2183 (38.847, -16.8277) -> (39.6304, -14.995)
  line L2184 (39.6304, -14.995) -> (39.8686, -14.9959)
  line L2185 (39.8686, -14.9959) -> (39.9151, -15.0968)
  line L2186 (39.9151, -15.0968) -> (38.9681, -17.3314)
  line L2187 (38.9681, -17.3314) -> (38.6852, -17.2809)
  line L2188 (38.6852, -17.2809) -> (37.7789, -15.0968)
  line L2189 (9.6819, 4.5673) -> (9.6819, 4.5673)
  line L2190 (40.641, -17.255) -> (40.6629, -15.0186)
  line L2191 (40.6629, -15.0186) -> (40.8101, -14.9641)
  line L2192 (40.8101, -14.9641) -> (42.0036, -14.9959)
  line L2193 (42.0036, -14.9959) -> (42.0474, -15.1011)
  line L2194 (42.0474, -15.1011) -> (41.8838, -15.1823)
  line L2195 (41.8838, -15.1823) -> (40.9792, -15.1823)
  line L2196 (40.9792, -15.1823) -> (40.9792, -16.055)
  line L2197 (40.9792, -16.055) -> (41.8317, -16.0868)
  line L2198 (41.8317, -16.0868) -> (41.8755, -16.1929)
  line L2199 (41.8755, -16.1929) -> (41.7119, -16.2732)
  line L2200 (41.7119, -16.2732) -> (40.9792, -16.2732)
  line L2201 (40.9792, -16.2732) -> (40.9792, -17.1459)
  line L2202 (40.9792, -17.1459) -> (42.0036, -17.1777)
  line L2203 (42.0036, -17.1777) -> (42.0474, -17.2829)
  line L2204 (42.0474, -17.2829) -> (41.8838, -17.3641)
  line L2205 (41.8838, -17.3641) -> (40.6903, -17.3323)
  line L2206 (40.6903, -17.3323) -> (40.641, -17.255)
  line L2207 (12.544, 2.4091) -> (12.544, 2.4091)
  line L2208 (43.2274, -15.5527) -> (43.2055, -17.3096)
  line L2209 (43.2055, -17.3096) -> (42.974, -17.35)
  line L2210 (42.974, -17.35) -> (42.8895, -17.2551)
  line L2211 (42.8895, -17.2551) -> (42.9114, -15.0186)
  line L2212 (42.9114, -15.0186) -> (43.1436, -14.9778)
  line L2213 (43.1436, -14.9778) -> (43.2077, -15.0204)
  line L2214 (43.2077, -15.0204) -> (44.4665, -16.7664)
  line L2215 (44.4665, -16.7664) -> (44.4884, -15.0186)
  line L2216 (44.4884, -15.0186) -> (44.7199, -14.9782)
  line L2217 (44.7199, -14.9782) -> (44.8044, -15.0731)
  line L2218 (44.8044, -15.0731) -> (44.7831, -17.3094)
  line L2219 (44.7831, -17.3094) -> (44.5516, -17.3496)
  line L2220 (44.5516, -17.3496) -> (44.4749, -17.2914)
  line L2221 (44.4749, -17.2914) -> (43.2274, -15.5527)
  line L2222 (15.1305, 4.1114) -> (15.1305, 4.1114)
  line L2223 (46.1779, -15.1823) -> (45.5921, -15.1395)
  line L2224 (45.5921, -15.1395) -> (45.5702, -15.0311)
  line L2225 (45.5702, -15.0311) -> (45.727, -14.9641)
  line L2226 (45.727, -14.9641) -> (47.0867, -14.9959)
  line L2227 (47.0867, -14.9959) -> (47.1306, -15.102)
  line L2228 (47.1306, -15.102) -> (46.967, -15.1823)
  line L2229 (46.967, -15.1823) -> (46.5161, -15.1823)
  line L2230 (46.5161, -15.1823) -> (46.4941, -17.3096)
  line L2231 (46.4941, -17.3096) -> (46.2624, -17.35)
  line L2232 (46.2624, -17.35) -> (46.1779, -17.255)
  line L2233 (46.1779, -17.255) -> (46.1779, -15.1823)
  line L2234 (18.0809, 4.4818) -> (18.0809, 4.4818)
  line L2235 (48.141, -17.255) -> (48.1629, -15.0186)
  line L2236 (48.1629, -15.0186) -> (48.3101, -14.9641)
  line L2237 (48.3101, -14.9641) -> (49.5036, -14.9959)
  line L2238 (49.5036, -14.9959) -> (49.5474, -15.1011)
  line L2239 (49.5474, -15.1011) -> (49.3838, -15.1823)
  line L2240 (49.3838, -15.1823) -> (48.4792, -15.1823)
  line L2241 (48.4792, -15.1823) -> (48.4792, -16.055)
  line L2242 (48.4792, -16.055) -> (49.3317, -16.0868)
  line L2243 (49.3317, -16.0868) -> (49.3755, -16.1929)
  line L2244 (49.3755, -16.1929) -> (49.2119, -16.2732)
  line L2245 (49.2119, -16.2732) -> (48.4792, -16.2732)
  line L2246 (48.4792, -16.2732) -> (48.4792, -17.1459)
  line L2247 (48.4792, -17.1459) -> (49.5036, -17.1777)
  line L2248 (49.5036, -17.1777) -> (49.5474, -17.2829)
  line L2249 (49.5474, -17.2829) -> (49.3838, -17.3641)
  line L2250 (49.3838, -17.3641) -> (48.1903, -17.3323)
  line L2251 (48.1903, -17.3323) -> (48.141, -17.255)
  line L2252 (20.044, 2.4091) -> (20.044, 2.4091)
  line L2253 (50.641, -17.255) -> (50.6629, -15.0186)
  line L2254 (50.6629, -15.0186) -> (50.8101, -14.9641)
  line L2255 (50.8101, -14.9641) -> (52.0036, -14.9959)
  line L2256 (52.0036, -14.9959) -> (52.0474, -15.1011)
  line L2257 (52.0474, -15.1011) -> (51.8838, -15.1823)
  line L2258 (51.8838, -15.1823) -> (50.9792, -15.1823)
  line L2259 (50.9792, -15.1823) -> (50.9792, -16.055)
  line L2260 (50.9792, -16.055) -> (51.8317, -16.0868)
  line L2261 (51.8317, -16.0868) -> (51.8755, -16.1929)
  line L2262 (51.8755, -16.1929) -> (51.7119, -16.2732)
  line L2263 (51.7119, -16.2732) -> (50.9792, -16.2732)
  line L2264 (50.9792, -16.2732) -> (50.9792, -17.1459)
  line L2265 (50.9792, -17.1459) -> (52.0036, -17.1777)
  line L2266 (52.0036, -17.1777) -> (52.0474, -17.2829)
  line L2267 (52.0474, -17.2829) -> (51.8838, -17.3641)
  line L2268 (51.8838, -17.3641) -> (50.6903, -17.3323)
  line L2269 (50.6903, -17.3323) -> (50.641, -17.255)
  line L2270 (22.544, 2.4091) -> (22.544, 2.4091)
  line L2271 (53.2274, -15.5527) -> (53.2055, -17.3096)
  line L2272 (53.2055, -17.3096) -> (52.974, -17.35)
  line L2273 (52.974, -17.35) -> (52.8895, -17.2551)
  line L2274 (52.8895, -17.2551) -> (52.9114, -15.0186)
  line L2275 (52.9114, -15.0186) -> (53.1436, -14.9778)
  line L2276 (53.1436, -14.9778) -> (53.2077, -15.0204)
  line L2277 (53.2077, -15.0204) -> (54.4665, -16.7664)
  line L2278 (54.4665, -16.7664) -> (54.4884, -15.0186)
  line L2279 (54.4884, -15.0186) -> (54.7199, -14.9782)
  line L2280 (54.7199, -14.9782) -> (54.8044, -15.0731)
  line L2281 (54.8044, -15.0731) -> (54.7831, -17.3094)
  line L2282 (54.7831, -17.3094) -> (54.5516, -17.3496)
  line L2283 (54.5516, -17.3496) -> (54.4749, -17.2914)
  line L2284 (54.4749, -17.2914) -> (53.2274, -15.5527)
  line L2285 (25.1305, 4.1114) -> (25.1305, 4.1114)
  line L2286 (55.641, -17.255) -> (55.6629, -15.0186)
  line L2287 (55.6629, -15.0186) -> (55.8101, -14.9641)
  line L2288 (55.8101, -14.9641) -> (57.0036, -14.9959)
  line L2289 (57.0036, -14.9959) -> (57.0474, -15.1011)
  line L2290 (57.0474, -15.1011) -> (56.8838, -15.1823)
  line L2291 (56.8838, -15.1823) -> (55.9792, -15.1823)
  line L2292 (55.9792, -15.1823) -> (55.9792, -16.055)
  line L2293 (55.9792, -16.055) -> (56.8317, -16.0868)
  line L2294 (56.8317, -16.0868) -> (56.8755, -16.1929)
  line L2295 (56.8755, -16.1929) -> (56.7119, -16.2732)
  line L2296 (56.7119, -16.2732) -> (55.9792, -16.2732)
  line L2297 (55.9792, -16.2732) -> (55.9792, -17.1459)
  line L2298 (55.9792, -17.1459) -> (57.0036, -17.1777)
  line L2299 (57.0036, -17.1777) -> (57.0474, -17.2829)
  line L2300 (57.0474, -17.2829) -> (56.8838, -17.3641)
  line L2301 (56.8838, -17.3641) -> (55.6903, -17.3323)
  line L2302 (55.6903, -17.3323) -> (55.641, -17.255)
  line L2303 (27.544, 2.4091) -> (27.544, 2.4091)
  line L2304 (58.8892, -17.1459) -> (59.1257, -17.0853)
  line L2305 (59.1257, -17.0853) -> (59.2648, -16.9696)
  line L2306 (59.2648, -16.9696) -> (59.2979, -16.8586)
  line L2307 (59.2979, -16.8586) -> (59.2942, -15.4341)
  line L2308 (59.2942, -15.4341) -> (59.239, -15.3285)
  line L2309 (59.239, -15.3285) -> (59.0712, -15.2203)
  line L2310 (59.0712, -15.2203) -> (58.847, -15.1823)
  line L2311 (58.847, -15.1823) -> (58.3961, -15.1823)
  line L2312 (58.3961, -15.1823) -> (58.3741, -17.3096)
  line L2313 (58.3741, -17.3096) -> (58.1424, -17.35)
  line L2314 (58.1424, -17.35) -> (58.0579, -17.255)
  line L2315 (58.0579, -17.255) -> (58.0798, -15.0186)
  line L2316 (58.0798, -15.0186) -> (58.227, -14.9641)
  line L2317 (58.227, -14.9641) -> (58.9533, -14.9682)
  line L2318 (58.9533, -14.9682) -> (59.2403, -15.0304)
  line L2319 (59.2403, -15.0304) -> (59.4756, -15.1646)
  line L2320 (59.4756, -15.1646) -> (59.5783, -15.2777)
  line L2321 (59.5783, -15.2777) -> (59.6296, -15.4046)
  line L2322 (59.6296, -15.4046) -> (59.6296, -16.9272)
  line L2323 (59.6296, -16.9272) -> (59.5783, -17.0536)
  line L2324 (59.5783, -17.0536) -> (59.4756, -17.166)
  line L2325 (59.4756, -17.166) -> (59.259, -17.293)
  line L2326 (59.259, -17.293) -> (59.0073, -17.3565)
  line L2327 (59.0073, -17.3565) -> (58.7562, -17.3096)
  line L2328 (58.7562, -17.3096) -> (58.7568, -17.2009)
  line L2329 (58.7568, -17.2009) -> (58.8892, -17.1459)
  line L2330 (30.7923, 2.5182) -> (30.7923, 2.5182)
  line L2331 (30.097, -17.6641) -> (60.097, -17.6641)
  line L2332 (60.097, -17.6641) -> (60.097, 15.3359)
  line L2333 (60.097, 15.3359) -> (30.097, 15.3359)
  line L2334 (30.097, 15.3359) -> (30.097, -17.6641)